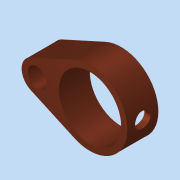
# Autodesk Inventor part: ShaftCollarMagnetMount
Saved by Autodesk Inventor 2017 (Build 210142000, 142)
## iProperties
Created: 2018-04-11
Part Number: ShaftCollarMagnetMount
Material: ABS Plastic
Document SubType Name: Modeling
Designer: Derek Wider
Density: 1.06 g/cm^3
Appearance: Copper - Satin
Author: Derek Wider
Autodesk Inventor part; units mm, degrees
ref_plane "XZ Plane" through (0, 0, 0) normal (0, 1, 0) x (-1, 0, 0)
ref_plane "XY Plane" through (0, 0, 0) normal (0, 0, 1) x (1, 0, 0)
sketch "Sketch2" plane through (0, 0, 0) normal (0, 0, 1) x (1, 0, 0)
  circle A0 centre (0, 0) radius 5.05
  circle A1 centre (-8.5, 0) radius 1.55
  circle A2 centre (-8.5, 0) radius 2.5
  circle A3 centre (0, 0) radius 6
  line L0 (-2.4706, 5.4677) -> (-9.5294, 2.2782)
  line L1 (-9.5294, -2.2782) -> (-2.4706, -5.4677)
  dimension "d0" = 10.1
  dimension "d1" = 3.1
  dimension "d2" = 5
  dimension "d3" = 12
  constraints: 5 tangent, 4 centre point, 4 end point, 4 point on circle, 3 coincident
  measures "d0" diameter of A0
  measures "d1" diameter of A1
  measures "d2" diameter of A2
  measures "d3" diameter of A3
extrude "Extrusion1" add sketch "Sketch2" along normal blind 5
extrude "Extrusion2" add sketch "Sketch2" along normal blind 3 contours A1
ref_plane "Work Plane1" through (6, 0, 0) normal (1, 0, 0) x (0, 1, 0)
sketch "Sketch3" plane through (6, 0, 0) normal (1, 0, 0) x (0, 1, 0)
  circle A0 centre (0, 2.5) radius 1.25
  line L0 (6, 0) -> (6, 5) construction
  point P0 (0, 0)
  point P1 (6, 2.5)
  dimension "d8" = 2.5
  constraints: 1 centre point, 1 horizontal alignment, 1 midpoint
  measures "d8" diameter of A0
extrude "Extrusion3" cut sketch "Sketch3" against normal blind 3
body "Solid1"
